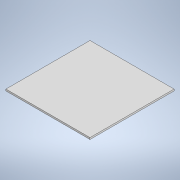
# Autodesk Inventor part: PisoDeEnsayoIgnorar
Saved by Autodesk Inventor 2021 (Build 250183000, 183)
## iProperties
Created: 2021-04-17
Part Number: PisoDeEnsayoIgnorar
Material: Generic
Document SubType Name: Modeling
Designer: GABRIEL LOL
Density: 1 g/cm^3
Appearance: Default
Author: GABRIEL LOL
Autodesk Inventor part; units mm, degrees
ref_plane "YZ Plane" through (0, 0, 0) normal (1, 0, 0) x (0, 1, 0)
ref_plane "XZ Plane" through (0, 0, 0) normal (0, 1, 0) x (-1, 0, 0)
ref_plane "XY Plane" through (0, 0, 0) normal (0, 0, 1) x (1, 0, 0)
sketch "Sketch1" plane through (0, 0, 0) normal (0, 1, 0) x (-1, 0, 0)
  line L0 (250, 250) -> (-250, 250)
  line L1 (-250, 250) -> (-250, -250)
  line L2 (-250, -250) -> (250, -250)
  line L3 (250, -250) -> (250, 250)
  line L4 (250, 250) -> (-250, -250) construction
  line L5 (-250, 250) -> (250, -250) construction
  point P0 (0, 0)
  dimension "d2" = 500
  dimension "d3" = 500
  constraints: 12 end point, 2 midpoint, 2 parallel, 1 horizontal, 1 perpendicular
  measures "d2" distance of L2.end L0.start
  measures "d3" distance of L0.start L0.end
extrude "Extrusion1" add sketch "Sketch1" along normal blind 10
body "Solid1"
